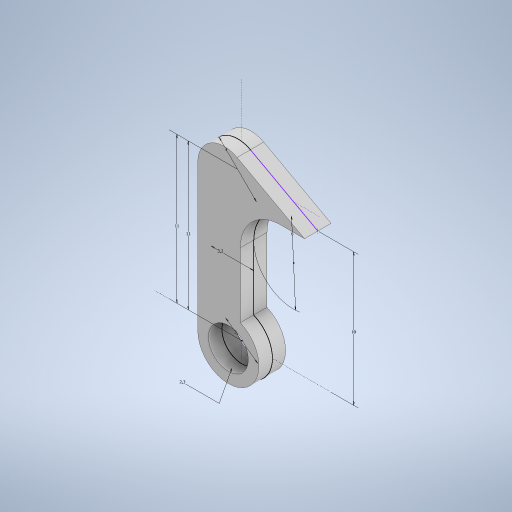
# Autodesk Inventor part: Hudson 1-62D
Saved by Autodesk Inventor 2024.2 (Build 282272000, 272)
## iProperties
Created: 2024-10-07
Part Number: Hudson 1-62D
Material: Genérico
Document SubType Name: Modeling
Designer: Monica Mora
Density: 1 g/cm^3
Appearance: Valor por defecto
Author: Monica Mora
Autodesk Inventor part; units mm, degrees
ref_plane "YZ Plane" through (0, 0, 0) normal (1, 0, 0) x (0, 1, 0)
ref_plane "XZ Plane" through (0, 0, 0) normal (0, 1, 0) x (-1, 0, 0)
ref_plane "XY Plane" through (0, 0, 0) normal (0, 0, 1) x (1, 0, 0)
sketch "Boceto1" plane through (0, 0, 0) normal (0, 0, 1) x (1, 0, 0)
  circle A0 centre (0, 0) radius 1.5
  circle A1 centre (0, 0) radius 2.3
  line L0 (-2.3, 0) -> (-2.3, 11)
  line L1 (0, -2.3) -> (0, 17.0308) construction
  circle A2 centre (-0.3, 11) radius 2
  line L2 (0.9, 7) -> (0.9, 2.1166)
  line L3 (-6.6108, 0) -> (6.6108, 0) construction
  arc A3 (3.9, 10) -> (0.9, 7) centre (3.9, 7) ccw
  line L4 (-2.4885, 11) -> (5.8935, 11) construction
  line L5 (0.8529, 10) -> (0.9, 10)
  line L6 (3.9, 10) -> (5.7216, 10)
  line L7 (0.656, 12.7567) -> (5.7248, 9.9983)
  dimension "d3" = 4
  dimension "d0" = 2.3
  dimension "d1" = 3
  dimension "d2" = 11
  dimension "d5" = 3.2
  dimension "d6" = 6
  dimension "d7" = 11
  dimension "d9" = 10
  constraints: 16 end point, 5 point on circle, 4 horizontal, 4 tangent, 3 centre point, 3 coincident, 3 vertical, 2 point on line, 1 midpoint, 4 other
  measures "d0" radius of A1
  measures "d1" diameter of A0
  measures "d2" distance of L0.start L0.end
  measures "d5" distance between parallel lines of L0 L2
  measures "d6" diameter of A3
  measures "d7" vertical distance of point (0, 0) point (-0.3, 11)
  measures "d9" distance between parallel lines of L3 L6
extrude "Extrusión1" add sketch "Boceto1" along normal mid plane 2
sketch "Boceto2" plane through (-2.3, 0, 1) normal (-1, 0, 0) x (0, 0, 1)
  line L0 (-1, 0) -> (-1, 11) construction
  line L1 (-2, 11) -> (0, 11) projected
  line L2 (-2, 0) -> (0, 0) projected
  line L3 (0, 11) -> (0, 0) projected
  line L4 (-2, 11) -> (0, 11) projected
  line L5 (-2, 0) -> (-2, 11) projected
  circle A0 centre (-1, 9) radius 0.5
  dimension "d12" = 1
  dimension "d13" = 9
  constraints: 2 end point, 1 centre point, 1 midpoint, 1 point on line
  measures "d12" diameter of A0
  measures "d13" distance from line of L2 A0.centre
hole "Agujero1" at (-2.3, 9, 0) direction (1, 0, 0) diameter 1 depth 2.3
